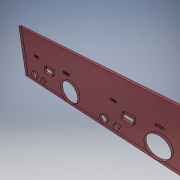
# Autodesk Inventor part: NavCom_plexi
Saved by Autodesk Inventor 2018 (Build 220112000, 112)
## iProperties
Created: 2017-02-12
Part Number: NavCom_plexi
Material: Sklo
Document SubType Name: Modeling
Designer: N
Density: 2.18 g/cm^3
Appearance: Čirá
Author: N
Autodesk Inventor part; units mm, degrees
ref_plane "YZ Plane" through (0, 0, 0) normal (1, 0, 0) x (0, 1, 0)
ref_plane "XZ Plane" through (0, 0, 0) normal (0, 1, 0) x (-1, 0, 0)
ref_plane "XY Plane" through (0, 0, 0) normal (0, 0, 1) x (1, 0, 0)
sketch "Náčrt1" plane through (0, 0, 0) normal (0, 0, 1) x (1, 0, 0)
  line L0 (0, 50.8) -> (172.72, 50.8)
  line L1 (172.72, 50.8) -> (172.72, 0)
  line L2 (172.72, 0) -> (0, 0)
  line L3 (0, 0) -> (0, 50.8)
  circle A0 centre (26.67, 6.35) radius 2.54
  circle A1 centre (13.97, 6.35) radius 3.81
  circle A2 centre (62.865, 11.43) radius 10.795
  circle A3 centre (114.3, 6.35) radius 2.54
  circle A4 centre (101.6, 6.35) radius 3.81
  circle A5 centre (150.495, 11.43) radius 10.795
  line L4 (31.75, 23.1775) -> (41.91, 23.1775)
  line L5 (41.91, 23.1775) -> (41.91, 17.4625)
  line L6 (41.91, 17.4625) -> (31.75, 17.4625)
  line L7 (31.75, 17.4625) -> (31.75, 23.1775)
  line L8 (119.38, 23.1775) -> (129.54, 23.1775)
  line L9 (129.54, 23.1775) -> (129.54, 17.4625)
  line L10 (129.54, 17.4625) -> (119.38, 17.4625)
  line L11 (119.38, 17.4625) -> (119.38, 23.1775)
  line L12 (19.05, 30.48) -> (24.9366, 30.48) construction
  line L13 (24.9366, 30.48) -> (24.9366, 27.8943) construction
  line L14 (24.9366, 27.8943) -> (19.05, 27.8943) construction
  line L15 (19.05, 27.8943) -> (19.05, 30.48) construction
  point P0 (57.15, 30.48)
  point P1 (146.05, 30.48)
  point P2 (107.95, 30.48)
  constraints: 24 end point, 6 centre point, 1 coincident, 9 other
extrude "Vysunutí2" add sketch "Náčrt1" along normal blind 2.54
sketch "Náčrt2" plane through (0, 0, 2.54) normal (0, 0, 1) x (1, 0, 0)
  line L0 (0, 50.8) -> (172.72, 50.8)
  line L1 (172.72, 50.8) -> (172.72, 0)
  line L2 (172.72, 0) -> (0, 0)
  line L3 (0, 0) -> (0, 50.8)
  circle A0 centre (26.67, 6.35) radius 2.54
  circle A1 centre (13.97, 6.35) radius 3.81
  circle A2 centre (62.865, 11.43) radius 10.795
  circle A3 centre (114.3, 6.35) radius 2.54
  circle A4 centre (101.6, 6.35) radius 3.81
  circle A5 centre (150.495, 11.43) radius 10.795
  line L4 (31.75, 23.1775) -> (41.91, 23.1775)
  line L5 (41.91, 23.1775) -> (41.91, 17.4625)
  line L6 (41.91, 17.4625) -> (31.75, 17.4625)
  line L7 (31.75, 17.4625) -> (31.75, 23.1775)
  line L8 (119.38, 23.1775) -> (129.54, 23.1775)
  line L9 (129.54, 23.1775) -> (129.54, 17.4625)
  line L10 (129.54, 17.4625) -> (119.38, 17.4625)
  line L11 (119.38, 17.4625) -> (119.38, 23.1775)
  line L12 (19.2546, 30.4371) -> (19.6677, 30.4371)
  line L13 (19.6677, 30.4371) -> (19.6677, 29.0829)
  spline S0 degree 2 poles (19.6677, 29.0829) (19.6677, 28.7672) (19.6833, 28.6717) knots 0 0 0 1 1 1
  spline S1 degree 2 poles (19.6833, 28.6717) (19.7106, 28.5061) (19.9171, 28.3249) (20.0866, 28.3249) knots 0 0 0 1 2 2 2
  spline S2 degree 2 poles (20.0866, 28.3249) (20.2289, 28.3249) (20.4101, 28.4535) (20.4763, 28.6795) (20.4763, 29.0537) knots 0 0 0 1 2 3 3 3
  line L14 (20.4763, 29.0537) -> (20.4763, 30.4371)
  line L15 (20.4763, 30.4371) -> (20.8894, 30.4371)
  line L16 (20.8894, 30.4371) -> (20.8894, 29.1238)
  spline S3 degree 2 poles (20.8894, 29.1238) (20.8894, 28.6211) (20.7823, 28.1729) (20.4062, 27.8943) (20.0964, 27.8943) knots 0 0 0 1 2 3 3 3
  spline S4 degree 2 poles (20.0964, 27.8943) (19.7768, 27.8943) (19.4163, 28.1242) (19.2546, 28.5431) (19.2546, 29.1043) knots 0 0 0 1 2 3 3 3
  line L17 (19.2546, 29.1043) -> (19.2546, 30.4371)
  line L18 (21.2226, 28.7516) -> (21.626, 28.8003)
  spline S5 degree 2 poles (21.626, 28.8003) (21.6942, 28.321) (22.0722, 28.321) knots 0 0 0 1 1 1
  spline S6 degree 2 poles (22.0722, 28.321) (22.2593, 28.321) (22.4736, 28.5178) (22.4736, 28.662) knots 0 0 0 1 2 2 2
  spline S7 degree 2 poles (22.4736, 28.662) (22.4736, 28.7477) (22.3996, 28.8666) (22.2456, 28.9426) (21.9514, 29.0342) knots 0 0 0 1 2 3 3 3
  spline S8 degree 2 poles (21.9514, 29.0342) (21.6864, 29.1141) (21.4409, 29.3011) (21.2967, 29.6051) (21.2967, 29.7805) knots 0 0 0 1 2 3 3 3
  spline S9 degree 2 poles (21.2967, 29.7805) (21.2967, 29.9851) (21.4818, 30.3124) (21.8111, 30.48) (22.0508, 30.48) knots 0 0 0 1 2 3 3 3
  spline S10 degree 2 poles (22.0508, 30.48) (22.4132, 30.48) (22.8185, 30.0864) (22.8302, 29.722) knots 0 0 0 1 2 2 2
  line L19 (22.8302, 29.722) -> (22.4152, 29.7006)
  spline S11 degree 2 poles (22.4152, 29.7006) (22.3879, 29.9032) (22.2067, 30.063) (22.041, 30.063) knots 0 0 0 1 2 2 2
  spline S12 degree 2 poles (22.041, 30.063) (21.8735, 30.063) (21.6922, 29.9227) (21.6922, 29.8194) knots 0 0 0 1 2 2 2
  spline S13 degree 2 poles (21.6922, 29.8194) (21.6922, 29.7181) (21.7741, 29.648) knots 0 0 0 1 1 1
  spline S14 degree 2 poles (21.7741, 29.648) (21.8559, 29.5778) (22.1501, 29.494) knots 0 0 0 1 1 1
  spline S15 degree 2 poles (22.1501, 29.494) (22.4619, 29.4044) (22.7406, 29.2037) (22.8867, 28.888) (22.8867, 28.6639) knots 0 0 0 1 2 3 3 3
  spline S16 degree 2 poles (22.8867, 28.6639) (22.8867, 28.3385) (22.4872, 27.8943) (22.0605, 27.8943) knots 0 0 0 1 2 2 2
  spline S17 degree 2 poles (22.0605, 27.8943) (21.3084, 27.8943) (21.2226, 28.7516) knots 0 0 0 1 1 1
  line L20 (23.2374, 27.9371) -> (23.2374, 30.4371)
  line L21 (23.2374, 30.4371) -> (24.7593, 30.4371)
  line L22 (24.7593, 30.4371) -> (24.7593, 30.0143)
  line L23 (24.7593, 30.0143) -> (23.6505, 30.0143)
  line L24 (23.6505, 30.0143) -> (23.6505, 29.459)
  line L25 (23.6505, 29.459) -> (24.6813, 29.459)
  line L26 (24.6813, 29.459) -> (24.6813, 29.0381)
  line L27 (24.6813, 29.0381) -> (23.6505, 29.0381)
  line L28 (23.6505, 29.0381) -> (23.6505, 28.36)
  line L29 (23.6505, 28.36) -> (24.7963, 28.36)
  line L30 (24.7963, 28.36) -> (24.7963, 27.9371)
  line L31 (24.7963, 27.9371) -> (23.2374, 27.9371)
  line L32 (57.2552, 28.7516) -> (57.6586, 28.8003)
  spline S18 degree 2 poles (57.6586, 28.8003) (57.7268, 28.321) (58.1048, 28.321) knots 0 0 0 1 1 1
  spline S19 degree 2 poles (58.1048, 28.321) (58.2919, 28.321) (58.5062, 28.5178) (58.5062, 28.662) knots 0 0 0 1 2 2 2
  spline S20 degree 2 poles (58.5062, 28.662) (58.5062, 28.7477) (58.4321, 28.8666) (58.2782, 28.9426) (57.984, 29.0342) knots 0 0 0 1 2 3 3 3
  spline S21 degree 2 poles (57.984, 29.0342) (57.719, 29.1141) (57.4735, 29.3011) (57.3293, 29.6051) (57.3293, 29.7805) knots 0 0 0 1 2 3 3 3
  spline S22 degree 2 poles (57.3293, 29.7805) (57.3293, 29.9851) (57.5144, 30.3124) (57.8437, 30.48) (58.0834, 30.48) knots 0 0 0 1 2 3 3 3
  spline S23 degree 2 poles (58.0834, 30.48) (58.4458, 30.48) (58.8511, 30.0864) (58.8628, 29.722) knots 0 0 0 1 2 2 2
  line L33 (58.8628, 29.722) -> (58.4477, 29.7006)
  spline S24 degree 2 poles (58.4477, 29.7006) (58.4205, 29.9032) (58.2392, 30.063) (58.0736, 30.063) knots 0 0 0 1 2 2 2
  spline S25 degree 2 poles (58.0736, 30.063) (57.906, 30.063) (57.7248, 29.9227) (57.7248, 29.8194) knots 0 0 0 1 2 2 2
  spline S26 degree 2 poles (57.7248, 29.8194) (57.7248, 29.7181) (57.8067, 29.648) knots 0 0 0 1 1 1
  spline S27 degree 2 poles (57.8067, 29.648) (57.8885, 29.5778) (58.1827, 29.494) knots 0 0 0 1 1 1
  spline S28 degree 2 poles (58.1827, 29.494) (58.4945, 29.4044) (58.7731, 29.2037) (58.9193, 28.888) (58.9193, 28.6639) knots 0 0 0 1 2 3 3 3
  spline S29 degree 2 poles (58.9193, 28.6639) (58.9193, 28.3385) (58.5198, 27.8943) (58.0931, 27.8943) knots 0 0 0 1 2 2 2
  spline S30 degree 2 poles (58.0931, 27.8943) (57.341, 27.8943) (57.2552, 28.7516) knots 0 0 0 1 1 1
  line L34 (59.7299, 27.9371) -> (59.7299, 30.0143)
  line L35 (59.7299, 30.0143) -> (59.1219, 30.0143)
  line L36 (59.1219, 30.0143) -> (59.1219, 30.4371)
  line L37 (59.1219, 30.4371) -> (60.7509, 30.4371)
  line L38 (60.7509, 30.4371) -> (60.7509, 30.0143)
  line L39 (60.7509, 30.0143) -> (60.143, 30.0143)
  line L40 (60.143, 30.0143) -> (60.143, 27.9371)
  line L41 (60.143, 27.9371) -> (59.7299, 27.9371)
  line L42 (61.0179, 30.4371) -> (61.8382, 30.4371)
  spline S31 degree 2 poles (61.8382, 30.4371) (62.1753, 30.4371) (62.4481, 30.3144) (62.6352, 30.0046) (62.6352, 29.8077) knots 0 0 0 1 2 3 3 3
  spline S32 degree 2 poles (62.6352, 29.8077) (62.6352, 29.6265) (62.4754, 29.3362) (62.3468, 29.2661) knots 0 0 0 1 2 2 2
  spline S33 degree 2 poles (62.3468, 29.2661) (62.528, 29.2017) (62.7346, 28.8861) (62.7346, 28.662) knots 0 0 0 1 2 2 2
  spline S34 degree 2 poles (62.7346, 28.662) (62.7346, 28.3892) (62.4715, 28.0131) (62.2922, 27.9683) knots 0 0 0 1 2 2 2
  spline S35 degree 2 poles (62.2922, 27.9683) (62.1695, 27.9371) (61.7155, 27.9371) knots 0 0 0 1 1 1
  line L43 (61.7155, 27.9371) -> (61.0179, 27.9371)
  line L44 (61.0179, 27.9371) -> (61.0179, 30.4371)
  line L45 (61.431, 29.0264) -> (61.431, 28.36)
  line L46 (61.431, 28.36) -> (61.8148, 28.36)
  spline S36 degree 2 poles (61.8148, 28.36) (62.0682, 28.36) (62.2104, 28.4126) (62.3078, 28.5665) (62.3078, 28.6873) knots 0 0 0 1 2 3 3 3
  spline S37 degree 2 poles (62.3078, 28.6873) (62.3078, 28.8081) (62.2045, 28.966) (62.0311, 29.0264) (61.7661, 29.0264) knots 0 0 0 1 2 3 3 3
  line L47 (61.7661, 29.0264) -> (61.431, 29.0264)
  line L48 (61.431, 30.0201) -> (61.431, 29.4434)
  line L49 (61.431, 29.4434) -> (61.7038, 29.4434)
  spline S38 degree 2 poles (61.7038, 29.4434) (61.9493, 29.4434) (62.0077, 29.4512) knots 0 0 0 1 1 1
  spline S39 degree 2 poles (62.0077, 29.4512) (62.113, 29.4687) (62.2318, 29.6129) (62.2318, 29.7376) knots 0 0 0 1 2 2 2
  spline S40 degree 2 poles (62.2318, 29.7376) (62.2318, 29.8487) (62.1344, 29.987) (61.9961, 30.0201) (61.6687, 30.0201) knots 0 0 0 1 2 3 3 3
  line L50 (61.6687, 30.0201) -> (61.431, 30.0201)
  line L51 (63.6231, 27.9371) -> (63.6231, 28.9894)
  line L52 (63.6231, 28.9894) -> (62.8729, 30.4371)
  line L53 (62.8729, 30.4371) -> (63.3581, 30.4371)
  line L54 (63.3581, 30.4371) -> (63.8394, 29.4492)
  line L55 (63.8394, 29.4492) -> (64.3148, 30.4371)
  line L56 (64.3148, 30.4371) -> (64.7903, 30.4371)
  line L57 (64.7903, 30.4371) -> (64.0362, 28.9874)
  line L58 (64.0362, 28.9874) -> (64.0362, 27.9371)
  line L59 (64.0362, 27.9371) -> (63.6231, 27.9371)
  line L60 (108.1546, 30.4371) -> (108.5677, 30.4371)
  line L61 (108.5677, 30.4371) -> (108.5677, 29.0829)
  spline S41 degree 2 poles (108.5677, 29.0829) (108.5677, 28.7672) (108.5833, 28.6717) knots 0 0 0 1 1 1
  spline S42 degree 2 poles (108.5833, 28.6717) (108.6106, 28.5061) (108.8171, 28.3249) (108.9866, 28.3249) knots 0 0 0 1 2 2 2
  spline S43 degree 2 poles (108.9866, 28.3249) (109.1289, 28.3249) (109.3101, 28.4535) (109.3763, 28.6795) (109.3763, 29.0537) knots 0 0 0 1 2 3 3 3
  line L62 (109.3763, 29.0537) -> (109.3763, 30.4371)
  line L63 (109.3763, 30.4371) -> (109.7894, 30.4371)
  line L64 (109.7894, 30.4371) -> (109.7894, 29.1238)
  spline S44 degree 2 poles (109.7894, 29.1238) (109.7894, 28.6211) (109.6823, 28.1729) (109.3062, 27.8943) (108.9964, 27.8943) knots 0 0 0 1 2 3 3 3
  spline S45 degree 2 poles (108.9964, 27.8943) (108.6768, 27.8943) (108.3163, 28.1242) (108.1546, 28.5431) (108.1546, 29.1043) knots 0 0 0 1 2 3 3 3
  line L65 (108.1546, 29.1043) -> (108.1546, 30.4371)
  line L66 (110.1226, 28.7516) -> (110.526, 28.8003)
  spline S46 degree 2 poles (110.526, 28.8003) (110.5942, 28.321) (110.9722, 28.321) knots 0 0 0 1 1 1
  spline S47 degree 2 poles (110.9722, 28.321) (111.1593, 28.321) (111.3736, 28.5178) (111.3736, 28.662) knots 0 0 0 1 2 2 2
  spline S48 degree 2 poles (111.3736, 28.662) (111.3736, 28.7477) (111.2996, 28.8666) (111.1456, 28.9426) (110.8514, 29.0342) knots 0 0 0 1 2 3 3 3
  spline S49 degree 2 poles (110.8514, 29.0342) (110.5864, 29.1141) (110.3409, 29.3011) (110.1967, 29.6051) (110.1967, 29.7805) knots 0 0 0 1 2 3 3 3
  spline S50 degree 2 poles (110.1967, 29.7805) (110.1967, 29.9851) (110.3818, 30.3124) (110.7111, 30.48) (110.9508, 30.48) knots 0 0 0 1 2 3 3 3
  spline S51 degree 2 poles (110.9508, 30.48) (111.3132, 30.48) (111.7185, 30.0864) (111.7302, 29.722) knots 0 0 0 1 2 2 2
  line L67 (111.7302, 29.722) -> (111.3152, 29.7006)
  spline S52 degree 2 poles (111.3152, 29.7006) (111.2879, 29.9032) (111.1067, 30.063) (110.941, 30.063) knots 0 0 0 1 2 2 2
  spline S53 degree 2 poles (110.941, 30.063) (110.7735, 30.063) (110.5922, 29.9227) (110.5922, 29.8194) knots 0 0 0 1 2 2 2
  spline S54 degree 2 poles (110.5922, 29.8194) (110.5922, 29.7181) (110.6741, 29.648) knots 0 0 0 1 1 1
  spline S55 degree 2 poles (110.6741, 29.648) (110.7559, 29.5778) (111.0501, 29.494) knots 0 0 0 1 1 1
  spline S56 degree 2 poles (111.0501, 29.494) (111.3619, 29.4044) (111.6406, 29.2037) (111.7867, 28.888) (111.7867, 28.6639) knots 0 0 0 1 2 3 3 3
  spline S57 degree 2 poles (111.7867, 28.6639) (111.7867, 28.3385) (111.3872, 27.8943) (110.9605, 27.8943) knots 0 0 0 1 2 2 2
  spline S58 degree 2 poles (110.9605, 27.8943) (110.2084, 27.8943) (110.1226, 28.7516) knots 0 0 0 1 1 1
  line L68 (112.1374, 27.9371) -> (112.1374, 30.4371)
  line L69 (112.1374, 30.4371) -> (113.6593, 30.4371)
  line L70 (113.6593, 30.4371) -> (113.6593, 30.0143)
  line L71 (113.6593, 30.0143) -> (112.5505, 30.0143)
  line L72 (112.5505, 30.0143) -> (112.5505, 29.459)
  line L73 (112.5505, 29.459) -> (113.5813, 29.459)
  line L74 (113.5813, 29.459) -> (113.5813, 29.0381)
  line L75 (113.5813, 29.0381) -> (112.5505, 29.0381)
  line L76 (112.5505, 29.0381) -> (112.5505, 28.36)
  line L77 (112.5505, 28.36) -> (113.6963, 28.36)
  line L78 (113.6963, 28.36) -> (113.6963, 27.9371)
  line L79 (113.6963, 27.9371) -> (112.1374, 27.9371)
  line L80 (146.1552, 28.7516) -> (146.5586, 28.8003)
  spline S59 degree 2 poles (146.5586, 28.8003) (146.6268, 28.321) (147.0048, 28.321) knots 0 0 0 1 1 1
  spline S60 degree 2 poles (147.0048, 28.321) (147.1919, 28.321) (147.4062, 28.5178) (147.4062, 28.662) knots 0 0 0 1 2 2 2
  spline S61 degree 2 poles (147.4062, 28.662) (147.4062, 28.7477) (147.3321, 28.8666) (147.1782, 28.9426) (146.884, 29.0342) knots 0 0 0 1 2 3 3 3
  spline S62 degree 2 poles (146.884, 29.0342) (146.619, 29.1141) (146.3735, 29.3011) (146.2293, 29.6051) (146.2293, 29.7805) knots 0 0 0 1 2 3 3 3
  spline S63 degree 2 poles (146.2293, 29.7805) (146.2293, 29.9851) (146.4144, 30.3124) (146.7437, 30.48) (146.9834, 30.48) knots 0 0 0 1 2 3 3 3
  spline S64 degree 2 poles (146.9834, 30.48) (147.3458, 30.48) (147.7511, 30.0864) (147.7628, 29.722) knots 0 0 0 1 2 2 2
  line L81 (147.7628, 29.722) -> (147.3477, 29.7006)
  spline S65 degree 2 poles (147.3477, 29.7006) (147.3205, 29.9032) (147.1392, 30.063) (146.9736, 30.063) knots 0 0 0 1 2 2 2
  spline S66 degree 2 poles (146.9736, 30.063) (146.806, 30.063) (146.6248, 29.9227) (146.6248, 29.8194) knots 0 0 0 1 2 2 2
  spline S67 degree 2 poles (146.6248, 29.8194) (146.6248, 29.7181) (146.7067, 29.648) knots 0 0 0 1 1 1
  spline S68 degree 2 poles (146.7067, 29.648) (146.7885, 29.5778) (147.0827, 29.494) knots 0 0 0 1 1 1
  spline S69 degree 2 poles (147.0827, 29.494) (147.3945, 29.4044) (147.6731, 29.2037) (147.8193, 28.888) (147.8193, 28.6639) knots 0 0 0 1 2 3 3 3
  spline S70 degree 2 poles (147.8193, 28.6639) (147.8193, 28.3385) (147.4198, 27.8943) (146.9931, 27.8943) knots 0 0 0 1 2 2 2
  spline S71 degree 2 poles (146.9931, 27.8943) (146.241, 27.8943) (146.1552, 28.7516) knots 0 0 0 1 1 1
  line L82 (148.6299, 27.9371) -> (148.6299, 30.0143)
  line L83 (148.6299, 30.0143) -> (148.0219, 30.0143)
  line L84 (148.0219, 30.0143) -> (148.0219, 30.4371)
  line L85 (148.0219, 30.4371) -> (149.6509, 30.4371)
  line L86 (149.6509, 30.4371) -> (149.6509, 30.0143)
  line L87 (149.6509, 30.0143) -> (149.043, 30.0143)
  line L88 (149.043, 30.0143) -> (149.043, 27.9371)
  line L89 (149.043, 27.9371) -> (148.6299, 27.9371)
  line L90 (149.9179, 30.4371) -> (150.7382, 30.4371)
  spline S72 degree 2 poles (150.7382, 30.4371) (151.0753, 30.4371) (151.3481, 30.3144) (151.5352, 30.0046) (151.5352, 29.8077) knots 0 0 0 1 2 3 3 3
  spline S73 degree 2 poles (151.5352, 29.8077) (151.5352, 29.6265) (151.3754, 29.3362) (151.2468, 29.2661) knots 0 0 0 1 2 2 2
  spline S74 degree 2 poles (151.2468, 29.2661) (151.428, 29.2017) (151.6346, 28.8861) (151.6346, 28.662) knots 0 0 0 1 2 2 2
  spline S75 degree 2 poles (151.6346, 28.662) (151.6346, 28.3892) (151.3715, 28.0131) (151.1922, 27.9683) knots 0 0 0 1 2 2 2
  spline S76 degree 2 poles (151.1922, 27.9683) (151.0695, 27.9371) (150.6155, 27.9371) knots 0 0 0 1 1 1
  line L91 (150.6155, 27.9371) -> (149.9179, 27.9371)
  line L92 (149.9179, 27.9371) -> (149.9179, 30.4371)
  line L93 (150.331, 29.0264) -> (150.331, 28.36)
  line L94 (150.331, 28.36) -> (150.7148, 28.36)
  spline S77 degree 2 poles (150.7148, 28.36) (150.9682, 28.36) (151.1104, 28.4126) (151.2078, 28.5665) (151.2078, 28.6873) knots 0 0 0 1 2 3 3 3
  spline S78 degree 2 poles (151.2078, 28.6873) (151.2078, 28.8081) (151.1045, 28.966) (150.9311, 29.0264) (150.6661, 29.0264) knots 0 0 0 1 2 3 3 3
  line L95 (150.6661, 29.0264) -> (150.331, 29.0264)
  line L96 (150.331, 30.0201) -> (150.331, 29.4434)
  line L97 (150.331, 29.4434) -> (150.6038, 29.4434)
  spline S79 degree 2 poles (150.6038, 29.4434) (150.8493, 29.4434) (150.9077, 29.4512) knots 0 0 0 1 1 1
  spline S80 degree 2 poles (150.9077, 29.4512) (151.013, 29.4687) (151.1318, 29.6129) (151.1318, 29.7376) knots 0 0 0 1 2 2 2
  spline S81 degree 2 poles (151.1318, 29.7376) (151.1318, 29.8487) (151.0344, 29.987) (150.8961, 30.0201) (150.5687, 30.0201) knots 0 0 0 1 2 3 3 3
  line L98 (150.5687, 30.0201) -> (150.331, 30.0201)
  line L99 (152.5231, 27.9371) -> (152.5231, 28.9894)
  line L100 (152.5231, 28.9894) -> (151.7729, 30.4371)
  line L101 (151.7729, 30.4371) -> (152.2581, 30.4371)
  line L102 (152.2581, 30.4371) -> (152.7394, 29.4492)
  line L103 (152.7394, 29.4492) -> (153.2148, 30.4371)
  line L104 (153.2148, 30.4371) -> (153.6903, 30.4371)
  line L105 (153.6903, 30.4371) -> (152.9362, 28.9874)
  line L106 (152.9362, 28.9874) -> (152.9362, 27.9371)
  line L107 (152.9362, 27.9371) -> (152.5231, 27.9371)
  point P0 (57.15, 30.48)
  point P1 (19.05, 30.48)
  point P2 (146.05, 30.48)
  point P3 (107.95, 30.48)
  constraints: 24 end point, 6 centre point, 4 other
extrude "Vysunutí3" add sketch "Náčrt2" along normal blind 0.0025 separate body contours L12 L13 S0 S1 S2 L14 L15 L16 S3 S4 L17 | L18 S5 S6 S7 S8 S9 S10 L19 S11 S12 S13 S14 S15 S16 S17 | L20 L21 L22 L23 L24 L25 L26 L27 L28 L29 L30 L31 | L32 S18 S19 S20 S21 S22 S23 L33 S24 S25 S26 S27 S28 S29 S30 | L34 L35 L36 L37 L38 L39 L40 L41 | L42 S31 S32 S33 S34 S35 L43 L44 | L51 L52 L53 L54 L55 L56 L57 L58 L59 | L60 L61 S41 S42 S43 L62 L63 L64 S44 S45 L65 | L66 S46 S47 S48 S49 S50 S51 L67 S52 S53 S54 S55 S56 S57 S58 | L68 L69 L70 L71 L72 L73 L74 L75 L76 L77 L78 L79 | L80 S59 S60 S61 S62 S63 S64 L81 S65 S66 S67 S68 S69 S70 S71 | L82 L83 L84 L85 L86 L87 L88 L89 | L90 S72 S73 S74 S75 S76 L91 L92 | L99 L100 L101 L102 L103 L104 L105 L106 L107
